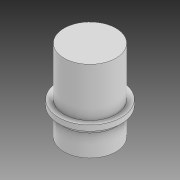
# Autodesk Inventor part: Stepper Shaft Extension
Saved by Autodesk Inventor 2020 (Build 240168000, 168)
## iProperties
Created: 2020-08-18
Part Number: Stepper Shaft Extension
Material: Generic
Document SubType Name: Modeling
Designer: DDeGo
Density: 1 g/cm^3
Appearance: Default
Author: DDeGo
Autodesk Inventor part; units mm, degrees
ref_plane "YZ Plane" through (0, 0, 0) normal (1, 0, 0) x (0, 1, 0)
ref_plane "XZ Plane" through (0, 0, 0) normal (0, 1, 0) x (-1, 0, 0)
ref_plane "XY Plane" through (0, 0, 0) normal (0, 0, 1) x (1, 0, 0)
sketch "Sketch1" plane through (0, 0, 0) normal (0, 0, 1) x (1, 0, 0)
  line L0 (0, 0) -> (0, 7.5)
  line L1 (0, 7.5) -> (2.4, 7.5)
  line L2 (2.4, 7.5) -> (2.4, 3)
  line L3 (2.4, 3) -> (2.9, 3)
  line L4 (2.9, 2) -> (2.4, 2) construction
  line L5 (2.4, 2) -> (2.4, 0)
  line L6 (2.4, 0) -> (0, 0)
  line L7 (2.4, 2) -> (2.9, 2.5)
  line L8 (2.9, 3) -> (2.9, 2.5)
  line L9 (2.9, 2.5) -> (2.9, 2) construction
  dimension "d0" = 2.4
  dimension "d1" = 2
  dimension "d2" = 1
  dimension "d3" = 4.5
  dimension "d7" = 45
  dimension "d8" = 0.5
  constraints: 20 end point, 7 perpendicular, 2 point on line, 1 vertical
  measures "d0" distance of L5.end L0.start
  measures "d1" distance of L4.end L5.end
  measures "d2" distance between parallel lines of L3 L4
  measures "d3" distance between parallel lines of L1 L3
  measures "d7" angle of L4 L7
  measures "d8" distance of L2.end L3.end
revolve "Revolution1" add sketch "Sketch1" angle 360 about axis through (0, 0, 0) along (0, 1, 0)
body "Solid1"
